Autodesk Fusion 360 part; units mm, degrees
(part 4 of 15)
  spline S55 degree 5 poles (25.1717, 7.6599) (25.182, 7.6631) (25.2028, 7.6691) (25.2341, 7.6774) (25.2761, 7.6871) (25.3292, 7.6971) (25.3826, 7.7058) (25.4363, 7.7136) (25.4901, 7.7209) (25.544, 7.7279) (25.598, 7.7346) (25.6521, 7.7408) (25.7063, 7.7465) (25.7606, 7.7514) (25.8152, 7.7557) (25.8698, 7.7594) (25.9246, 7.7625) (25.9795, 7.7651) (26.0345, 7.7673) (26.0895, 7.7692) (26.1446, 7.7706) (26.1998, 7.7717) (26.2551, 7.7724) (26.3104, 7.7726) (26.3659, 7.7725) (26.4214, 7.7719) (26.4769, 7.7709) (26.5326, 7.7695) (26.5883, 7.7678) (26.644, 7.7657) (26.6999, 7.7633) (26.7557, 7.7606) (26.8117, 7.7575) (26.8676, 7.754) (26.9237, 7.7502) (26.9797, 7.7461) (27.0359, 7.7417) (27.092, 7.7369) (27.1483, 7.7318) (27.2045, 7.7264) (27.2608, 7.7206) (27.3172, 7.7146) (27.3735, 7.7083) (27.4299, 7.7016) (27.4864, 7.6947) (27.5429, 7.6874) (27.5994, 7.6799) (27.6559, 7.672) (27.7125, 7.6639) (27.7691, 7.6555) (27.8257, 7.6468) (27.8824, 7.6378) (27.9391, 7.6285) (27.9958, 7.6189) (28.0525, 7.6091) (28.1093, 7.599) (28.166, 7.5886) (28.2228, 7.5779) (28.2796, 7.567) (28.3365, 7.5558) (28.3933, 7.5443) (28.4502, 7.5326) (28.5071, 7.5206) (28.564, 7.5083) (28.6209, 7.4958) (28.6778, 7.483) (28.7347, 7.47) (28.7917, 7.4567) (28.8486, 7.4431) (28.9056, 7.4293) (28.9625, 7.4152) (29.0081, 7.4038) (29.0423, 7.3951) (29.0651, 7.3892) (29.0765, 7.3863) knots 0 0 0 0 0 0 0.01428571 0.02857143 0.04285714 0.05714286 0.07142857 0.08571429 0.1 0.11428571 0.12857143 0.14285714 0.15714286 0.17142857 0.18571429 0.2 0.21428571 0.22857143 0.24285714 0.25714286 0.27142857 0.28571429 0.3 0.31428571 0.32857143 0.34285714 0.35714286 0.37142857 0.38571429 0.4 0.41428571 0.42857143 0.44285714 0.45714286 0.47142857 0.48571429 0.5 0.51428571 0.52857143 0.54285714 0.55714286 0.57142857 0.58571429 0.6 0.61428571 0.62857143 0.64285714 0.65714286 0.67142857 0.68571429 0.7 0.71428571 0.72857143 0.74285714 0.75714286 0.77142857 0.78571429 0.8 0.81428571 0.82857143 0.84285714 0.85714286 0.87142857 0.88571429 0.9 0.91428571 0.92857143 0.94285714 0.95714286 0.97142857 0.98571429 1 1 1 1 1 1
  line L55 (25.1717, 7.6599) -> (24.5734, 7.4779)
  circle A57 centre (0, 0) radius 20
  dimension "d90" = 40
  constraint concentric A0 A57
  measures "d90" diameter of A57
extrude "Extrude3'" add sketch "Sketch4" along normal blind 40 contours A0 | A57 bodies 9 in component "Spur Gear 28 teeth"
hole "Hole1" at (0, 20, -27.403) direction (0, -1, 0) diameter 8 end through all bodies 9 in component "Spur Gear 28 teeth"
pattern_circular "C-Pattern2" count 3 over 360 about axis through (0, 0, -40) along (0, 0, -1) of "Hole1" in component "Spur Gear 28 teeth"
sketch "Base Circle (3)" plane through (0, 0, 0) normal (0, 0, 1) x (1, 0, 0) in component "Spur Gear 88 teeth"
  circle A0 centre (0, 0) radius 68.5488
  circle A1 centre (0, 0) radius 10
extrude "Extrude1''''" add sketch "Base Circle (3)" along normal blind 20 separate body makes body 10 in component "Spur Gear 88 teeth"
sketch "Gear Tooth (3)" plane through (0, 0, 0) normal (0, 0, 1) x (1, 0, 0) in component "Spur Gear 88 teeth"
  spline S0 degree 5 poles (66.1189, -2.1665) (66.1359, -2.1663) (66.1698, -2.166) (66.2208, -2.1651) (66.2887, -2.1631) (66.3736, -2.1595) (66.4585, -2.1546) (66.5434, -2.1486) (66.6283, -2.1414) (66.7132, -2.1332) (66.7981, -2.1241) (66.8829, -2.1141) (66.9678, -2.1035) (67.0526, -2.0922) (67.1374, -2.0802) (67.2222, -2.0677) (67.3069, -2.0546) (67.3917, -2.0409) (67.4764, -2.0267) (67.561, -2.0118) (67.6457, -1.9964) (67.7303, -1.9805) (67.8149, -1.964) (67.8995, -1.9471) (67.984, -1.9297) (68.0685, -1.9118) (68.153, -1.8935) (68.2374, -1.8747) (68.3218, -1.8554) (68.4062, -1.8357) (68.4905, -1.8156) (68.5748, -1.795) (68.6591, -1.774) (68.7433, -1.7526) (68.8275, -1.7308) (68.9117, -1.7086) (68.9958, -1.686) (69.0799, -1.6631) (69.164, -1.6397) (69.248, -1.6159) (69.332, -1.5918) (69.4159, -1.5673) (69.4999, -1.5425) (69.5837, -1.5172) (69.6675, -1.4917) (69.7513, -1.4657) (69.8351, -1.4394) (69.9188, -1.4128) (70.0025, -1.3858) (70.0861, -1.3585) (70.1697, -1.3308) (70.2532, -1.3028) (70.3367, -1.2745) (70.4201, -1.2458) (70.5036, -1.2169) (70.5869, -1.1876) (70.6703, -1.1579) (70.7535, -1.128) (70.8368, -1.0977) (70.92, -1.0672) (71.0031, -1.0363) (71.0862, -1.0051) (71.1692, -0.9736) (71.2522, -0.9418) (71.3352, -0.9097) (71.4181, -0.8773) (71.501, -0.8446) (71.5838, -0.8116) (71.6666, -0.7783) (71.7493, -0.7447) (71.832, -0.7108) (71.8981, -0.6835) (71.9476, -0.6629) (71.9806, -0.649) (71.9971, -0.6421) knots 0 0 0 0 0 0 0.01428571 0.02857143 0.04285714 0.05714286 0.07142857 0.08571429 0.1 0.11428571 0.12857143 0.14285714 0.15714286 0.17142857 0.18571429 0.2 0.21428571 0.22857143 0.24285714 0.25714286 0.27142857 0.28571429 0.3 0.31428571 0.32857143 0.34285714 0.35714286 0.37142857 0.38571429 0.4 0.41428571 0.42857143 0.44285714 0.45714286 0.47142857 0.48571429 0.5 0.51428571 0.52857143 0.54285714 0.55714286 0.57142857 0.58571429 0.6 0.61428571 0.62857143 0.64285714 0.65714286 0.67142857 0.68571429 0.7 0.71428571 0.72857143 0.74285714 0.75714286 0.77142857 0.78571429 0.8 0.81428571 0.82857143 0.84285714 0.85714286 0.87142857 0.88571429 0.9 0.91428571 0.92857143 0.94285714 0.95714286 0.97142857 0.98571429 1 1 1 1 1 1
  spline S1 degree 5 poles (66.1189, 2.1665) (66.1359, 2.1663) (66.1698, 2.166) (66.2208, 2.1651) (66.2887, 2.1631) (66.3736, 2.1595) (66.4585, 2.1546) (66.5434, 2.1486) (66.6283, 2.1414) (66.7132, 2.1332) (66.7981, 2.1241) (66.8829, 2.1141) (66.9678, 2.1035) (67.0526, 2.0922) (67.1374, 2.0802) (67.2222, 2.0677) (67.3069, 2.0546) (67.3917, 2.0409) (67.4764, 2.0267) (67.561, 2.0118) (67.6457, 1.9964) (67.7303, 1.9805) (67.8149, 1.964) (67.8995, 1.9471) (67.984, 1.9297) (68.0685, 1.9118) (68.153, 1.8935) (68.2374, 1.8747) (68.3218, 1.8554) (68.4062, 1.8357) (68.4905, 1.8156) (68.5748, 1.795) (68.6591, 1.774) (68.7433, 1.7526) (68.8275, 1.7308) (68.9117, 1.7086) (68.9958, 1.686) (69.0799, 1.6631) (69.164, 1.6397) (69.248, 1.6159) (69.332, 1.5918) (69.4159, 1.5673) (69.4999, 1.5425) (69.5837, 1.5172) (69.6675, 1.4917) (69.7513, 1.4657) (69.8351, 1.4394) (69.9188, 1.4128) (70.0025, 1.3858) (70.0861, 1.3585) (70.1697, 1.3308) (70.2532, 1.3028) (70.3367, 1.2745) (70.4201, 1.2458) (70.5036, 1.2169) (70.5869, 1.1876) (70.6703, 1.1579) (70.7535, 1.128) (70.8368, 1.0977) (70.92, 1.0672) (71.0031, 1.0363) (71.0862, 1.0051) (71.1692, 0.9736) (71.2522, 0.9418) (71.3352, 0.9097) (71.4181, 0.8773) (71.501, 0.8446) (71.5838, 0.8116) (71.6666, 0.7783) (71.7493, 0.7447) (71.832, 0.7108) (71.8981, 0.6835) (71.9476, 0.6629) (71.9806, 0.649) (71.9971, 0.6421) knots 0 0 0 0 0 0 0.01428571 0.02857143 0.04285714 0.05714286 0.07142857 0.08571429 0.1 0.11428571 0.12857143 0.14285714 0.15714286 0.17142857 0.18571429 0.2 0.21428571 0.22857143 0.24285714 0.25714286 0.27142857 0.28571429 0.3 0.31428571 0.32857143 0.34285714 0.35714286 0.37142857 0.38571429 0.4 0.41428571 0.42857143 0.44285714 0.45714286 0.47142857 0.48571429 0.5 0.51428571 0.52857143 0.54285714 0.55714286 0.57142857 0.58571429 0.6 0.61428571 0.62857143 0.64285714 0.65714286 0.67142857 0.68571429 0.7 0.71428571 0.72857143 0.74285714 0.75714286 0.77142857 0.78571429 0.8 0.81428571 0.82857143 0.84285714 0.85714286 0.87142857 0.88571429 0.9 0.91428571 0.92857143 0.94285714 0.95714286 0.97142857 0.98571429 1 1 1 1 1 1
  arc A0 (71.9971, -0.6421) -> (71.9971, 0.6421) centre (0, 0) ccw
  line L0 (66.1189, 2.1665) -> (66.1189, -2.1665)
  point P0 (66.5372, -2.1488)
  point P1 (66.9564, -2.1048)
  point P2 (67.376, -2.0434)
  point P3 (67.796, -1.9676)
  point P4 (68.2162, -1.8793)
  point P5 (68.6366, -1.7796)
  point P6 (69.057, -1.6693)
  point P7 (69.4775, -1.549)
  point P8 (69.8979, -1.4194)
  point P9 (70.3182, -1.2807)
  point P10 (70.7383, -1.1334)
  point P11 (71.1582, -0.9777)
  point P12 (71.5778, -0.8139)
  point P13 (66.5372, 2.1488)
  point P14 (66.9564, 2.1048)
  point P15 (67.376, 2.0434)
  point P16 (67.796, 1.9676)
  point P17 (68.2162, 1.8793)
  point P18 (68.6366, 1.7796)
  point P19 (69.057, 1.6693)
  point P20 (69.4775, 1.549)
  point P21 (69.8979, 1.4194)
  point P22 (70.3182, 1.2807)
  point P23 (70.7383, 1.1334)
  point P24 (71.1582, 0.9777)
  point P25 (71.5778, 0.8139)
extrude "Extrude2''''" add sketch "Gear Tooth (3)" along normal blind 20 bodies 10 in component "Spur Gear 88 teeth"
pattern_circular "C-Pattern1''" count 88 over 360 about axis through (0, 0, 0) along (0, 0, 1) of "Extrude2''''" in component "Spur Gear 88 teeth"
sketch "Diametrial Pitch Circle (3)" plane through (0, 0, 0) normal (0, 0, 1) x (1, 0, 0) in component "Spur Gear 88 teeth"
  circle A0 centre (0, 0) radius 70.4 construction
scale "Scale1" factor 1.03 about (35.5272, 58.6239, 20) bodies 10 in component "Spur Gear 88 teeth"
sketch "Sketch1 (3)" plane through (0, 173.8907, 0) normal (0, -1, 0) x (1, 0, 0) in component "Base2"
  arc A0 (68.5305, -56.0481) -> (68.5775, -54.7308) centre (-2.0032, -52.8695) ccw
  spline S0 degree 5 poles (68.5775, -54.7308) (68.5878, -54.7283) (68.6154, -54.7216) (68.6604, -54.7105) (68.7228, -54.6949) (68.8024, -54.6747) (68.8892, -54.6522) (68.9759, -54.6294) (69.0625, -54.6061) (69.1491, -54.5824) (69.2357, -54.5584) (69.3222, -54.5339) (69.4087, -54.5091) (69.4952, -54.4838) (69.5816, -54.4582) (69.668, -54.4322) (69.7544, -54.4059) (69.8407, -54.3792) (69.9269, -54.3521) (70.0131, -54.3247) (70.0993, -54.2969) (70.1854, -54.2687) (70.2715, -54.2402) (70.3576, -54.2114) (70.4436, -54.1822) (70.5295, -54.1527) (70.6155, -54.1228) (70.7013, -54.0927) (70.7871, -54.0621) (70.8729, -54.0313) (70.9587, -54.0001) (71.0443, -53.9686) (71.13, -53.9368) (71.2156, -53.9047) (71.3011, -53.8723) (71.3866, -53.8395) (71.472, -53.8064) (71.5574, -53.7731) (71.6428, -53.7394) (71.7281, -53.7054) (71.8133, -53.6711) (71.8985, -53.6365) (71.9837, -53.6016) (72.0518, -53.5735) (72.1028, -53.5522) (72.1368, -53.538) (72.1538, -53.5309) knots 0.405839 0.405839 0.405839 0.405839 0.405839 0.405839 0.414286 0.428571 0.442857 0.457143 0.471429 0.485714 0.5 0.514286 0.528571 0.542857 0.557143 0.571429 0.585714 0.6 0.614286 0.628571 0.642857 0.657143 0.671429 0.685714 0.7 0.714286 0.728571 0.742857 0.757143 0.771429 0.785714 0.8 0.814286 0.828571 0.842857 0.857143 0.871429 0.885714 0.9 0.914286 0.928571 0.942857 0.957143 0.971429 0.985714 1 1 1 1 1 1
  arc A1 (72.1538, -53.5309) -> (72.1538, -52.2081) centre (-2.0032, -52.8695) ccw
  spline S1 degree 5 poles (72.1538, -52.2081) (72.1368, -52.201) (72.1028, -52.1867) (72.0518, -52.1655) (71.9837, -52.1373) (71.8985, -52.1025) (71.8133, -52.0679) (71.7281, -52.0336) (71.6428, -51.9996) (71.5574, -51.9659) (71.472, -51.9325) (71.3866, -51.8995) (71.3011, -51.8667) (71.2156, -51.8343) (71.13, -51.8021) (71.0443, -51.7703) (70.9587, -51.7388) (70.8729, -51.7077) (70.7871, -51.6768) (70.7013, -51.6463) (70.6155, -51.6161) (70.5295, -51.5863) (70.4436, -51.5567) (70.3576, -51.5276) (70.2715, -51.4987) (70.1854, -51.4702) (70.0993, -51.4421) (70.0131, -51.4143) (69.9269, -51.3869) (69.8407, -51.3598) (69.7544, -51.3331) (69.668, -51.3067) (69.5816, -51.2807) (69.4952, -51.2551) (69.4087, -51.2299) (69.3222, -51.2051) (69.2357, -51.1806) (69.1491, -51.1565) (69.0625, -51.1329) (68.9759, -51.1096) (68.8892, -51.0867) (68.8024, -51.0643) (68.7228, -51.044) (68.6604, -51.0285) (68.6154, -51.0174) (68.5878, -51.0107) (68.5775, -51.0082) knots -1 -1 -1 -1 -1 -1 -0.985714 -0.971429 -0.957143 -0.942857 -0.928571 -0.914286 -0.9 -0.885714 -0.871429 -0.857143 -0.842857 -0.828571 -0.814286 -0.8 -0.785714 -0.771429 -0.757143 -0.742857 -0.728571 -0.714286 -0.7 -0.685714 -0.671429 -0.657143 -0.642857 -0.628571 -0.614286 -0.6 -0.585714 -0.571429 -0.557143 -0.542857 -0.528571 -0.514286 -0.5 -0.485714 -0.471429 -0.457143 -0.442857 -0.428571 -0.414286 -0.405839 -0.405839 -0.405839 -0.405839 -0.405839 -0.405839
  arc A2 (68.5775, -51.0082) -> (68.5305, -49.6909) centre (-2.0032, -52.8695) ccw
  spline S2 degree 5 poles (68.5305, -49.6909) (68.5405, -49.6877) (68.5676, -49.679) (68.6117, -49.6647) (68.6728, -49.6447) (68.7508, -49.6189) (68.8357, -49.5903) (68.9206, -49.5613) (69.0053, -49.5319) (69.09, -49.5021) (69.1747, -49.4719) (69.2593, -49.4414) (69.3438, -49.4104) (69.4282, -49.3791) (69.5126, -49.3474) (69.5969, -49.3153) (69.6811, -49.2828) (69.7653, -49.25) (69.8494, -49.2169) (69.9335, -49.1834) (70.0174, -49.1495) (70.1013, -49.1153) (70.1852, -49.0807) (70.2689, -49.0458) (70.3526, -49.0106) (70.4363, -48.975) (70.5198, -48.9391) (70.6033, -48.9029) (70.6868, -48.8663) (70.7701, -48.8294) (70.8534, -48.7922) (70.9366, -48.7547) (71.0198, -48.7169) (71.1029, -48.6787) (71.1859, -48.6402) (71.2688, -48.6015) (71.3517, -48.5624) (71.4345, -48.523) (71.5172, -48.4833) (71.5999, -48.4433) (71.6825, -48.403) (71.765, -48.3625) (71.8474, -48.3216) (71.9133, -48.2887) (71.9627, -48.2638) (71.9956, -48.2472) (72.0121, -48.2389) knots 0.405839 0.405839 0.405839 0.405839 0.405839 0.405839 0.414286 0.428571 0.442857 0.457143 0.471429 0.485714 0.5 0.514286 0.528571 0.542857 0.557143 0.571429 0.585714 0.6 0.614286 0.628571 0.642857 0.657143 0.671429 0.685714 0.7 0.714286 0.728571 0.742857 0.757143 0.771429 0.785714 0.8 0.814286 0.828571 0.842857 0.857143 0.871429 0.885714 0.9 0.914286 0.928571 0.942857 0.957143 0.971429 0.985714 1 1 1 1 1 1
  arc A3 (72.0121, -48.2389) -> (71.9177, -46.9195) centre (-2.0032, -52.8695) ccw
  spline S3 degree 5 poles (71.9177, -46.9195) (71.9002, -46.9136) (71.8653, -46.9018) (71.8129, -46.8843) (71.743, -46.861) (71.6555, -46.8323) (71.5681, -46.8039) (71.4806, -46.7758) (71.3931, -46.748) (71.3056, -46.7204) (71.218, -46.6932) (71.1304, -46.6664) (71.0428, -46.6398) (70.9552, -46.6135) (70.8675, -46.5876) (70.7798, -46.562) (70.6921, -46.5367) (70.6044, -46.5117) (70.5166, -46.487) (70.4288, -46.4627) (70.341, -46.4387) (70.2532, -46.4151) (70.1653, -46.3918) (70.0775, -46.3688) (69.9896, -46.3462) (69.9017, -46.3239) (69.8138, -46.302) (69.7258, -46.2804) (69.6379, -46.2592) (69.5499, -46.2384) (69.4619, -46.2179) (69.3739, -46.1977) (69.2859, -46.178) (69.1979, -46.1586) (69.1098, -46.1396) (69.0218, -46.121) (68.9337, -46.1028) (68.8456, -46.0849) (68.7576, -46.0675) (68.6695, -46.0505) (68.5814, -46.0339) (68.4932, -46.0177) (68.4123, -46.0032) (68.349, -45.9921) (68.3034, -45.9843) (68.2753, -45.9795) (68.2649, -45.9777) knots -1 -1 -1 -1 -1 -1 -0.985714 -0.971429 -0.957143 -0.942857 -0.928571 -0.914286 -0.9 -0.885714 -0.871429 -0.857143 -0.842857 -0.828571 -0.814286 -0.8 -0.785714 -0.771429 -0.757143 -0.742857 -0.728571 -0.714286 -0.7 -0.685714 -0.671429 -0.657143 -0.642857 -0.628571 -0.614286 -0.6 -0.585714 -0.571429 -0.557143 -0.542857 -0.528571 -0.514286 -0.5 -0.485714 -0.471429 -0.457143 -0.442857 -0.428571 -0.414286 -0.405839 -0.405839 -0.405839 -0.405839 -0.405839 -0.405839
  arc A4 (68.2649, -45.9777) -> (68.124, -44.6672) centre (-2.0032, -52.8695) ccw
  spline S4 degree 5 poles (68.124, -44.6672) (68.1338, -44.6632) (68.1602, -44.6526) (68.2032, -44.6353) (68.2627, -44.611) (68.3386, -44.5796) (68.4213, -44.5451) (68.5038, -44.5101) (68.5863, -44.4747) (68.6687, -44.439) (68.7509, -44.4028) (68.8331, -44.3663) (68.9152, -44.3294) (68.9972, -44.2921) (69.0791, -44.2545) (69.1609, -44.2165) (69.2426, -44.1781) (69.3242, -44.1394) (69.4058, -44.1003) (69.4872, -44.0608) (69.5686, -44.0211) (69.6498, -43.981) (69.731, -43.9405) (69.812, -43.8997) (69.893, -43.8586) (69.9739, -43.8172) (70.0547, -43.7754) (70.1354, -43.7333) (70.216, -43.6909) (70.2965, -43.6481) (70.3769, -43.6051) (70.4572, -43.5617) (70.5375, -43.518) (70.6176, -43.4741) (70.6977, -43.4298) (70.7776, -43.3852) (70.8575, -43.3403) (70.9373, -43.2951) (71.017, -43.2496) (71.0966, -43.2038) (71.1761, -43.1577) (71.2555, -43.1114) (71.3348, -43.0647) (71.3982, -43.0272) (71.4457, -42.9989) (71.4773, -42.98) (71.4932, -42.9705) knots 0.405839 0.405839 0.405839 0.405839 0.405839 0.405839 0.414286 0.428571 0.442857 0.457143 0.471429 0.485714 0.5 0.514286 0.528571 0.542857 0.557143 0.571429 0.585714 0.6 0.614286 0.628571 0.642857 0.657143 0.671429 0.685714 0.7 0.714286 0.728571 0.742857 0.757143 0.771429 0.785714 0.8 0.814286 0.828571 0.842857 0.857143 0.871429 0.885714 0.9 0.914286 0.928571 0.942857 0.957143 0.971429 0.985714 1 1 1 1 1 1
  arc A5 (71.4932, -42.9705) -> (71.3049, -41.6612) centre (-2.0032, -52.8695) ccw
  spline S5 degree 5 poles (71.3049, -41.6612) (71.2871, -41.6565) (71.2514, -41.6473) (71.1978, -41.6335) (71.1264, -41.6154) (71.0372, -41.5929) (70.9479, -41.5708) (70.8587, -41.549) (70.7694, -41.5275) (70.6801, -41.5063) (70.5908, -41.4854) (70.5016, -41.4649) (70.4123, -41.4446) (70.323, -41.4247) (70.2337, -41.4051) (70.1444, -41.3858) (70.0551, -41.3668) (69.9658, -41.3481) (69.8765, -41.3298) (69.7872, -41.3118) (69.6979, -41.2942) (69.6086, -41.2768) (69.5194, -41.2599) (69.4301, -41.2432) (69.3408, -41.2269) (69.2515, -41.211) (69.1623, -41.1954) (69.073, -41.1801) (68.9838, -41.1652) (68.8945, -41.1507) (68.8053, -41.1365) (68.7161, -41.1227) (68.6269, -41.1093) (68.5377, -41.0963) (68.4485, -41.0836) (68.3594, -41.0713) (68.2702, -41.0594) (68.1811, -41.0479) (68.092, -41.0368) (68.0029, -41.0261) (67.9139, -41.0158) (67.8248, -41.006) (67.7431, -40.9973) (67.6792, -40.9907) (67.633, -40.9862) (67.6047, -40.9834) (67.5942, -40.9824) knots -1 -1 -1 -1 -1 -1 -0.985714 -0.971429 -0.957143 -0.942857 -0.928571 -0.914286 -0.9 -0.885714 -0.871429 -0.857143 -0.842857 -0.828571 -0.814286 -0.8 -0.785714 -0.771429 -0.757143 -0.742857 -0.728571 -0.714286 -0.7 -0.685714 -0.671429 -0.657143 -0.642857 -0.628571 -0.614286 -0.6 -0.585714 -0.571429 -0.557143 -0.542857 -0.528571 -0.514286 -0.5 -0.485714 -0.471429 -0.457143 -0.442857 -0.428571 -0.414286 -0.405839 -0.405839 -0.405839 -0.405839 -0.405839 -0.405839
  arc A6 (67.5942, -40.9824) -> (67.3602, -39.6853) centre (-2.0032, -52.8695) ccw
  spline S6 degree 5 poles (67.3602, -39.6853) (67.3697, -39.6806) (67.3952, -39.6682) (67.4369, -39.6478) (67.4945, -39.6193) (67.568, -39.5826) (67.648, -39.5422) (67.7279, -39.5015) (67.8076, -39.4603) (67.8872, -39.4188) (67.9667, -39.3769) (68.046, -39.3346) (68.1253, -39.2919) (68.2044, -39.2489) (68.2834, -39.2055) (68.3623, -39.1617) (68.4411, -39.1176) (68.5197, -39.0732) (68.5982, -39.0284) (68.6767, -38.9832) (68.755, -38.9377) (68.8331, -38.8919) (68.9112, -38.8458) (68.9892, -38.7993) (69.067, -38.7525) (69.1447, -38.7054) (69.2223, -38.658) (69.2998, -38.6102) (69.3772, -38.5622) (69.4544, -38.5138) (69.5316, -38.4651) (69.6086, -38.4162) (69.6855, -38.3669) (69.7623, -38.3173) (69.839, -38.2674) (69.9156, -38.2172) (69.9921, -38.1667) (70.0684, -38.116) (70.1447, -38.0649) (70.2208, -38.0136) (70.2968, -37.9619) (70.3727, -37.91) (70.4485, -37.8578) (70.509, -37.8159) (70.5544, -37.7842) (70.5846, -37.7631) (70.5997, -37.7525) knots 0.405839 0.405839 0.405839 0.405839 0.405839 0.405839 0.414286 0.428571 0.442857 0.457143 0.471429 0.485714 0.5 0.514286 0.528571 0.542857 0.557143 0.571429 0.585714 0.6 0.614286 0.628571 0.642857 0.657143 0.671429 0.685714 0.7 0.714286 0.728571 0.742857 0.757143 0.771429 0.785714 0.8 0.814286 0.828571 0.842857 0.857143 0.871429 0.885714 0.9 0.914286 0.928571 0.942857 0.957143 0.971429 0.985714 1 1 1 1 1 1
  arc A7 (70.5997, -37.7525) -> (70.3185, -36.46) centre (-2.0032, -52.8695) ccw
  spline S7 degree 5 poles (70.3185, -36.46) (70.3004, -36.4566) (70.2641, -36.45) (70.2097, -36.4401) (70.1372, -36.427) (70.0466, -36.411) (69.956, -36.3953) (69.8654, -36.38) (69.7748, -36.3649) (69.6843, -36.3501) (69.5937, -36.3356) (69.5032, -36.3215) (69.4127, -36.3077) (69.3222, -36.2941) (69.2318, -36.2809) (69.1413, -36.2681) (69.0509, -36.2555) (68.9605, -36.2433) (68.8701, -36.2314) (68.7798, -36.2198) (68.6895, -36.2085) (68.5992, -36.1976) (68.5089, -36.1871) (68.4187, -36.1768) (68.3285, -36.167) (68.2383, -36.1574) (68.1481, -36.1482) (68.058, -36.1394) (67.9679, -36.1309) (67.8779, -36.1228) (67.7879, -36.115) (67.6979, -36.1076) (67.608, -36.1006) (67.5181, -36.0939) (67.4282, -36.0877) (67.3384, -36.0818) (67.2487, -36.0763) (67.159, -36.0712) (67.0693, -36.0664) (66.9797, -36.0621) (66.8901, -36.0582) (66.8006, -36.0547) (66.7184, -36.0519) (66.6542, -36.0499) (66.6079, -36.0487) (66.5794, -36.0479) (66.5689, -36.0477) knots -1 -1 -1 -1 -1 -1 -0.985714 -0.971429 -0.957143 -0.942857 -0.928571 -0.914286 -0.9 -0.885714 -0.871429 -0.857143 -0.842857 -0.828571 -0.814286 -0.8 -0.785714 -0.771429 -0.757143 -0.742857 -0.728571 -0.714286 -0.7 -0.685714 -0.671429 -0.657143 -0.642857 -0.628571 -0.614286 -0.6 -0.585714 -0.571429 -0.557143 -0.542857 -0.528571 -0.514286 -0.5 -0.485714 -0.471429 -0.457143 -0.442857 -0.428571 -0.414286 -0.405839 -0.405839 -0.405839 -0.405839 -0.405839 -0.405839
  arc A8 (66.5689, -36.0477) -> (66.2429, -34.7705) centre (-2.0032, -52.8695) ccw
  spline S8 degree 5 poles (66.2429, -34.7705) (66.252, -34.7652) (66.2767, -34.751) (66.3167, -34.7277) (66.3721, -34.6952) (66.4429, -34.6533) (66.5198, -34.6073) (66.5965, -34.561) (66.6731, -34.5142) (66.7496, -34.4671) (66.8258, -34.4196) (66.902, -34.3718) (66.978, -34.3236) (67.0538, -34.275) (67.1295, -34.2261) (67.2051, -34.1768) (67.2805, -34.1272) (67.3558, -34.0773) (67.4309, -34.027) (67.5059, -33.9764) (67.5808, -33.9254) (67.6555, -33.8741) (67.7301, -33.8226) (67.8045, -33.7706) (67.8788, -33.7184) (67.953, -33.6659) (68.027, -33.613) (68.1009, -33.5599) (68.1746, -33.5064) (68.2482, -33.4527) (68.3217, -33.3986) (68.3951, -33.3442) (68.4683, -33.2896) (68.5413, -33.2347) (68.6143, -33.1794) (68.6871, -33.1239) (68.7598, -33.0681) (68.8323, -33.012) (68.9047, -32.9557) (68.977, -32.899) (69.0491, -32.8421) (69.1211, -32.7849) (69.193, -32.7274) (69.2504, -32.6812) (69.2934, -32.6465) (69.322, -32.6233) (69.3363, -32.6116) knots 0.405839 0.405839 0.405839 0.405839 0.405839 0.405839 0.414286 0.428571 0.442857 0.457143 0.471429 0.485714 0.5 0.514286 0.528571 0.542857 0.557143 0.571429 0.585714 0.6 0.614286 0.628571 0.642857 0.657143 0.671429 0.685714 0.7 0.714286 0.728571 0.742857 0.757143 0.771429 0.785714 0.8 0.814286 0.828571 0.842857 0.857143 0.871429 0.885714 0.9 0.914286 0.928571 0.942857 0.957143 0.971429 0.985714 1 1 1 1 1 1
  arc A9 (69.3363, -32.6116) -> (68.9636, -31.3424) centre (-2.0032, -52.8695) ccw
  spline S9 degree 5 poles (68.9636, -31.3424) (68.9453, -31.3404) (68.9087, -31.3363) (68.8537, -31.3303) (68.7804, -31.3225) (68.6889, -31.313) (68.5974, -31.3038) (68.506, -31.2949) (68.4145, -31.2863) (68.3232, -31.2781) (68.2318, -31.2701) (68.1405, -31.2624) (68.0493, -31.2551) (67.958, -31.2481) (67.8669, -31.2414) (67.7757, -31.235) (67.6846, -31.2289) (67.5936, -31.2231) (67.5026, -31.2177) (67.4117, -31.2126) (67.3208, -31.2078) (67.2299, -31.2034) (67.1391, -31.1993) (67.0484, -31.1955) (66.9577, -31.1921) (66.8671, -31.189) (66.7765, -31.1863) (66.686, -31.1839) (66.5955, -31.1819) (66.5052, -31.1802) (66.4148, -31.1789) (66.3246, -31.1779) (66.2343, -31.1773) (66.1442, -31.1771) (66.0541, -31.1772) (65.9641, -31.1778) (65.8742, -31.1787) (65.7844, -31.18) (65.6946, -31.1817) (65.6049, -31.1838) (65.5153, -31.1862) (65.4257, -31.1891) (65.3436, -31.1922) (65.2794, -31.1948) (65.2331, -31.1969) (65.2047, -31.1982) (65.1941, -31.1987) knots -1 -1 -1 -1 -1 -1 -0.985714 -0.971429 -0.957143 -0.942857 -0.928571 -0.914286 -0.9 -0.885714 -0.871429 -0.857143 -0.842857 -0.828571 -0.814286 -0.8 -0.785714 -0.771429 -0.757143 -0.742857 -0.728571 -0.714286 -0.7 -0.685714 -0.671429 -0.657143 -0.642857 -0.628571 -0.614286 -0.6 -0.585714 -0.571429 -0.557143 -0.542857 -0.528571 -0.514286 -0.5 -0.485714 -0.471429 -0.457143 -0.442857 -0.428571 -0.414286 -0.405839 -0.405839 -0.405839 -0.405839 -0.405839 -0.405839
  arc A10 (65.1941, -31.1987) -> (64.7778, -29.948) centre (-2.0032, -52.8695) ccw
  spline S10 degree 5 poles (64.7778, -29.948) (64.7866, -29.9421) (64.8101, -29.9261) (64.8484, -29.9) (64.9014, -29.8636) (64.969, -29.8168) (65.0424, -29.7655) (65.1156, -29.7138) (65.1887, -29.6617) (65.2616, -29.6092) (65.3343, -29.5564) (65.4068, -29.5033) (65.4792, -29.4498) (65.5514, -29.3959) (65.6234, -29.3417) (65.6953, -29.2872) (65.7669, -29.2323) (65.8385, -29.1771) (65.9098, -29.1216) (65.981, -29.0658) (66.052, -29.0096) (66.1229, -28.9531) (66.1936, -28.8964) (66.2642, -28.8393) (66.3345, -28.7819) (66.4048, -28.7242) (66.4748, -28.6662) (66.5447, -28.6079) (66.6145, -28.5493) (66.6841, -28.4905) (66.7535, -28.4313) (66.8228, -28.3718) (66.8919, -28.3121) (66.9609, -28.2521) (67.0297, -28.1918) (67.0983, -28.1312) (67.1668, -28.0704) (67.2352, -28.0093) (67.3034, -27.9479) (67.3714, -27.8862) (67.4393, -27.8243) (67.5071, -27.7621) (67.5747, -27.6997) (67.6286, -27.6495) (67.669, -27.6118) (67.6959, -27.5866) (67.7093, -27.5739) knots 0.405839 0.405839 0.405839 0.405839 0.405839 0.405839 0.414286 0.428571 0.442857 0.457143 0.471429 0.485714 0.5 0.514286 0.528571 0.542857 0.557143 0.571429 0.585714 0.6 0.614286 0.628571 0.642857 0.657143 0.671429 0.685714 0.7 0.714286 0.728571 0.742857 0.757143 0.771429 0.785714 0.8 0.814286 0.828571 0.842857 0.857143 0.871429 0.885714 0.9 0.914286 0.928571 0.942857 0.957143 0.971429 0.985714 1 1 1 1 1 1
  arc A11 (67.7093, -27.5739) -> (67.2471, -26.3346) centre (-2.0032, -52.8695) ccw
  spline S11 degree 5 poles (67.2471, -26.3346) (67.2287, -26.3338) (67.1918, -26.3324) (67.1366, -26.3303) (67.0629, -26.3277) (66.971, -26.3248) (66.8791, -26.3222) (66.7872, -26.3198) (66.6954, -26.3178) (66.6037, -26.3161) (66.512, -26.3146) (66.4204, -26.3135) (66.3288, -26.3127) (66.2373, -26.3122) (66.1459, -26.312) (66.0545, -26.3121) (65.9633, -26.3126) (65.872, -26.3133) (65.7809, -26.3144) (65.6898, -26.3158) (65.5988, -26.3175) (65.5079, -26.3196) (65.417, -26.322) (65.3263, -26.3247) (65.2356, -26.3277) (65.1449, -26.3311) (65.0544, -26.3348) (64.964, -26.3389) (64.8736, -26.3433) (64.7833, -26.3481) (64.6931, -26.3532) (64.603, -26.3587) (64.513, -26.3646) (64.4231, -26.3708) (64.3332, -26.3774) (64.2435, -26.3843) (64.1539, -26.3916) (64.0643, -26.3993) (63.9749, -26.4074) (63.8856, -26.4159) (63.7964, -26.4248) (63.7073, -26.4341) (63.6255, -26.4429) (63.5617, -26.4502) (63.5157, -26.4555) (63.4874, -26.4588) (63.4769, -26.4601) knots -1 -1 -1 -1 -1 -1 -0.985714 -0.971429 -0.957143 -0.942857 -0.928571 -0.914286 -0.9 -0.885714 -0.871429 -0.857143 -0.842857 -0.828571 -0.814286 -0.8 -0.785714 -0.771429 -0.757143 -0.742857 -0.728571 -0.714286 -0.7 -0.685714 -0.671429 -0.657143 -0.642857 -0.628571 -0.614286 -0.6 -0.585714 -0.571429 -0.557143 -0.542857 -0.528571 -0.514286 -0.5 -0.485714 -0.471429 -0.457143 -0.442857 -0.428571 -0.414286 -0.405839 -0.405839 -0.405839 -0.405839 -0.405839 -0.405839
  arc A12 (63.4769, -26.4601) -> (62.9725, -25.2423) centre (-2.0032, -52.8695) ccw
  spline S12 degree 5 poles (62.9725, -25.2423) (62.9808, -25.2358) (63.0031, -25.2181) (63.0395, -25.1894) (63.0897, -25.1493) (63.1538, -25.0978) (63.2233, -25.0414) (63.2927, -24.9846) (63.3619, -24.9274) (63.4308, -24.8699) (63.4996, -24.812) (63.5681, -24.7538) (63.6365, -24.6953) (63.7047, -24.6364) (63.7726, -24.5772) (63.8404, -24.5177) (63.908, -24.4579) (63.9754, -24.3977) (64.0426, -24.3373) (64.1097, -24.2765) (64.1765, -24.2154) (64.2432, -24.154) (64.3096, -24.0923) (64.3759, -24.0304) (64.442, -23.9681) (64.508, -23.9055) (64.5737, -23.8427) (64.6393, -23.7796) (64.7047, -23.7162) (64.7699, -23.6525) (64.8349, -23.5885) (64.8998, -23.5243) (64.9645, -23.4598) (65.029, -23.395) (65.0933, -23.3299) (65.1575, -23.2646) (65.2215, -23.199) (65.2853, -23.1332) (65.3489, -23.0671) (65.4124, -23.0008) (65.4757, -22.9341) (65.5388, -22.8673) (65.6018, -22.8002) (65.652, -22.7463) (65.6896, -22.7058) (65.7147, -22.6787) (65.7272, -22.6651) knots 0.405839 0.405839 0.405839 0.405839 0.405839 0.405839 0.414286 0.428571 0.442857 0.457143 0.471429 0.485714 0.5 0.514286 0.528571 0.542857 0.557143 0.571429 0.585714 0.6 0.614286 0.628571 0.642857 0.657143 0.671429 0.685714 0.7 0.714286 0.728571 0.742857 0.757143 0.771429 0.785714 0.8 0.814286 0.828571 0.842857 0.857143 0.871429 0.885714 0.9 0.914286 0.928571 0.942857 0.957143 0.971429 0.985714 1 1 1 1 1 1
  arc A13 (65.7272, -22.6651) -> (65.1777, -21.4619) centre (-2.0032, -52.8695) ccw
  spline S13 degree 5 poles (65.1777, -21.4619) (65.1592, -21.4625) (65.1224, -21.4637) (65.0671, -21.4656) (64.9935, -21.4682) (64.9016, -21.4719) (64.8097, -21.4758) (64.7179, -21.48) (64.6262, -21.4845) (64.5346, -21.4894) (64.443, -21.4945) (64.3515, -21.4999) (64.2602, -21.5056) (64.1689, -21.5116) (64.0777, -21.518) (63.9866, -21.5246) (63.8955, -21.5315) (63.8046, -21.5388) (63.7138, -21.5464) (63.623, -21.5543) (63.5324, -21.5625) (63.4418, -21.571) (63.3514, -21.5799) (63.261, -21.5891) (63.1708, -21.5986) (63.0806, -21.6084) (62.9906, -21.6186) (62.9007, -21.6291) (62.8108, -21.64) (62.7211, -21.6512) (62.6315, -21.6627) (62.542, -21.6746) (62.4527, -21.6869) (62.3634, -21.6995) (62.2743, -21.7125) (62.1853, -21.7258) (62.0964, -21.7395) (62.0076, -21.7536) (61.919, -21.768) (61.8305, -21.7829) (61.7422, -21.7981) (61.654, -21.8137) (61.5731, -21.8284) (61.5099, -21.8401) (61.4644, -21.8487) (61.4364, -21.8541) (61.4261, -21.8561) knots -1 -1 -1 -1 -1 -1 -0.985714 -0.971429 -0.957143 -0.942857 -0.928571 -0.914286 -0.9 -0.885714 -0.871429 -0.857143 -0.842857 -0.828571 -0.814286 -0.8 -0.785714 -0.771429 -0.757143 -0.742857 -0.728571 -0.714286 -0.7 -0.685714 -0.671429 -0.657143 -0.642857 -0.628571 -0.614286 -0.6 -0.585714 -0.571429 -0.557143 -0.542857 -0.528571 -0.514286 -0.5 -0.485714 -0.471429 -0.457143 -0.442857 -0.428571 -0.414286 -0.405839 -0.405839 -0.405839 -0.405839 -0.405839 -0.405839
  arc A14 (61.4261, -21.8561) -> (60.836, -20.6774) centre (-2.0032, -52.8695) ccw
  spline S14 degree 5 poles (60.836, -20.6774) (60.8439, -20.6703) (60.8649, -20.6511) (60.8991, -20.6198) (60.9463, -20.5763) (61.0066, -20.5203) (61.0719, -20.4591) (61.137, -20.3975) (61.202, -20.3355) (61.2666, -20.2732) (61.3311, -20.2106) (61.3953, -20.1477) (61.4593, -20.0844) (61.5231, -20.0208) (61.5867, -19.9569) (61.6501, -19.8927) (61.7132, -19.8282) (61.7762, -19.7634) (61.8389, -19.6983) (61.9014, -19.6329) (61.9637, -19.5672) (62.0258, -19.5012) (62.0877, -19.435) (62.1494, -19.3684) (62.2109, -19.3016) (62.2722, -19.2345) (62.3333, -19.1671) (62.3942, -19.0995) (62.4549, -19.0316) (62.5154, -18.9634) (62.5757, -18.8949) (62.6359, -18.8262) (62.6958, -18.7573) (62.7555, -18.6881) (62.815, -18.6186) (62.8744, -18.5489) (62.9335, -18.4789) (62.9925, -18.4087) (63.0512, -18.3382) (63.1098, -18.2675) (63.1682, -18.1965) (63.2264, -18.1253) (63.2844, -18.0539) (63.3307, -17.9966) (63.3653, -17.9535) (63.3883, -17.9247) (63.3998, -17.9103) knots 0.405839 0.405839 0.405839 0.405839 0.405839 0.405839 0.414286 0.428571 0.442857 0.457143 0.471429 0.485714 0.5 0.514286 0.528571 0.542857 0.557143 0.571429 0.585714 0.6 0.614286 0.628571 0.642857 0.657143 0.671429 0.685714 0.7 0.714286 0.728571 0.742857 0.757143 0.771429 0.785714 0.8 0.814286 0.828571 0.842857 0.857143 0.871429 0.885714 0.9 0.914286 0.928571 0.942857 0.957143 0.971429 0.985714 1 1 1 1 1 1
  arc A15 (63.3998, -17.9103) -> (62.7659, -16.7493) centre (-2.0032, -52.8695) ccw
  spline S15 degree 5 poles (62.7659, -16.7493) (62.7476, -16.7512) (62.7109, -16.755) (62.6559, -16.7608) (62.5827, -16.7687) (62.4912, -16.7789) (62.3999, -16.7894) (62.3086, -16.8002) (62.2174, -16.8112) (62.1264, -16.8226) (62.0354, -16.8342) (61.9446, -16.8461) (61.8539, -16.8583) (61.7632, -16.8709) (61.6727, -16.8837) (61.5823, -16.8968) (61.492, -16.9102) (61.4018, -16.924) (61.3118, -16.938) (61.2218, -16.9523) (61.132, -16.967) (61.0423, -16.982) (60.9527, -16.9973) (60.8632, -17.0129) (60.7739, -17.0288) (60.6847, -17.0451) (60.5956, -17.0616) (60.5066, -17.0785) (60.4178, -17.0958) (60.3291, -17.1134) (60.2406, -17.1313) (60.1522, -17.1495) (60.0639, -17.1681) (59.9758, -17.1871) (59.8878, -17.2063) (59.8, -17.226) (59.7123, -17.246) (59.6248, -17.2664) (59.5374, -17.2871) (59.4502, -17.3082) (59.3631, -17.3297) (59.2763, -17.3516) (59.1966, -17.372) (59.1345, -17.3882) (59.0897, -17.4) (59.0622, -17.4074) (59.052, -17.4101) knots -1 -1 -1 -1 -1 -1 -0.985714 -0.971429 -0.957143 -0.942857 -0.928571 -0.914286 -0.9 -0.885714 -0.871429 -0.857143 -0.842857 -0.828571 -0.814286 -0.8 -0.785714 -0.771429 -0.757143 -0.742857 -0.728571 -0.714286 -0.7 -0.685714 -0.671429 -0.657143 -0.642857 -0.628571 -0.614286 -0.6 -0.585714 -0.571429 -0.557143 -0.542857 -0.528571 -0.514286 -0.5 -0.485714 -0.471429 -0.457143 -0.442857 -0.428571 -0.414286 -0.405839 -0.405839 -0.405839 -0.405839 -0.405839 -0.405839
  arc A16 (59.052, -17.4101) -> (58.3794, -16.2765) centre (-2.0032, -52.8695) ccw
  spline S16 degree 5 poles (58.3794, -16.2765) (58.3867, -16.2688) (58.4063, -16.2482) (58.4381, -16.2146) (58.4822, -16.1678) (58.5383, -16.1077) (58.5991, -16.0419) (58.6596, -15.9758) (58.72, -15.9094) (58.78, -15.8427) (58.8399, -15.7756) (58.8994, -15.7082) (58.9588, -15.6406) (59.0179, -15.5726) (59.0767, -15.5043) (59.1354, -15.4358) (59.1937, -15.3669) (59.2519, -15.2978) (59.3098, -15.2284) (59.3675, -15.1587) (59.425, -15.0887) (59.4822, -15.0185) (59.5393, -14.9479) (59.5961, -14.8772) (59.6526, -14.8061) (59.709, -14.7348) (59.7651, -14.6633) (59.821, -14.5914) (59.8767, -14.5194) (59.9322, -14.4471) (59.9875, -14.3745) (60.0425, -14.3017) (60.0974, -14.2286) (60.152, -14.1553) (60.2065, -14.0818) (60.2607, -14.008) (60.3147, -13.934) (60.3685, -13.8597) (60.4221, -13.7852) (60.4754, -13.7105) (60.5286, -13.6356) (60.5816, -13.5604) (60.6344, -13.485) (60.6764, -13.4246) (60.7079, -13.3791) (60.7288, -13.3487) (60.7392, -13.3335) knots 0.405839 0.405839 0.405839 0.405839 0.405839 0.405839 0.414286 0.428571 0.442857 0.457143 0.471429 0.485714 0.5 0.514286 0.528571 0.542857 0.557143 0.571429 0.585714 0.6 0.614286 0.628571 0.642857 0.657143 0.671429 0.685714 0.7 0.714286 0.728571 0.742857 0.757143 0.771429 0.785714 0.8 0.814286 0.828571 0.842857 0.857143 0.871429 0.885714 0.9 0.914286 0.928571 0.942857 0.957143 0.971429 0.985714 1 1 1 1 1 1
  arc A17 (60.7392, -13.3335) -> (60.0241, -12.2208) centre (-2.0032, -52.8695) ccw
  spline S17 degree 5 poles (60.0241, -12.2208) (60.0059, -12.224) (59.9696, -12.2304) (59.9152, -12.2401) (59.8427, -12.2532) (59.7522, -12.2699) (59.6618, -12.2869) (59.5716, -12.3041) (59.4815, -12.3216) (59.3914, -12.3394) (59.3016, -12.3575) (59.2118, -12.3759) (59.1222, -12.3946) (59.0327, -12.4135) (58.9433, -12.4328) (58.854, -12.4523) (58.7649, -12.4721) (58.676, -12.4923) (58.5871, -12.5127) (58.4984, -12.5334) (58.4099, -12.5545) (58.3215, -12.5758) (58.2332, -12.5974) (58.1451, -12.6194) (58.0571, -12.6417) (57.9693, -12.6642) (57.8816, -12.6871) (57.7941, -12.7103) (57.7067, -12.7339) (57.6195, -12.7577) (57.5325, -12.7819) (57.4456, -12.8064) (57.3589, -12.8313) (57.2723, -12.8564) (57.1859, -12.882) (57.0997, -12.9078) (57.0137, -12.934) (56.9278, -12.9606) (56.8422, -12.9875) (56.7567, -13.0148) (56.6714, -13.0424) (56.5863, -13.0704) (56.5083, -13.0965) (56.4475, -13.1171) (56.4037, -13.1321) (56.3768, -13.1414) (56.3668, -13.1448) knots -1 -1 -1 -1 -1 -1 -0.985714 -0.971429 -0.957143 -0.942857 -0.928571 -0.914286 -0.9 -0.885714 -0.871429 -0.857143 -0.842857 -0.828571 -0.814286 -0.8 -0.785714 -0.771429 -0.757143 -0.742857 -0.728571 -0.714286 -0.7 -0.685714 -0.671429 -0.657143 -0.642857 -0.628571 -0.614286 -0.6 -0.585714 -0.571429 -0.557143 -0.542857 -0.528571 -0.514286 -0.5 -0.485714 -0.471429 -0.457143 -0.442857 -0.428571 -0.414286 -0.405839 -0.405839 -0.405839 -0.405839 -0.405839 -0.405839
  arc A18 (56.3668, -13.1448) -> (55.615, -12.0621) centre (-2.0032, -52.8695) ccw
  spline S18 degree 5 poles (55.615, -12.0621) (55.6217, -12.0539) (55.6398, -12.032) (55.6692, -11.9961) (55.7098, -11.9463) (55.7614, -11.8824) (55.8174, -11.8124) (55.8731, -11.7422) (55.9285, -11.6716) (55.9837, -11.6008) (56.0386, -11.5296) (56.0932, -11.4582) (56.1476, -11.3864) (56.2017, -11.3144) (56.2555, -11.2421) (56.3091, -11.1696) (56.3624, -11.0967) (56.4155, -11.0236) (56.4683, -10.9502) (56.5209, -10.8766) (56.5732, -10.8027) (56.6253, -10.7286) (56.6772, -10.6542) (56.7288, -10.5795) (56.7801, -10.5046) (56.8313, -10.4295) (56.8821, -10.3541) (56.9328, -10.2785) (56.9832, -10.2026) (57.0334, -10.1265) (57.0833, -10.0502) (57.1331, -9.9736) (57.1826, -9.8969) (57.2318, -9.8198) (57.2809, -9.7426) (57.3297, -9.6651) (57.3783, -9.5875) (57.4266, -9.5096) (57.4748, -9.4315) (57.5227, -9.3531) (57.5704, -9.2746) (57.6179, -9.1958) (57.6651, -9.1169) (57.7027, -9.0535) (57.7309, -9.006) (57.7496, -8.9742) (57.7589, -8.9583) knots 0.405839 0.405839 0.405839 0.405839 0.405839 0.405839 0.414286 0.428571 0.442857 0.457143 0.471429 0.485714 0.5 0.514286 0.528571 0.542857 0.557143 0.571429 0.585714 0.6 0.614286 0.628571 0.642857 0.657143 0.671429 0.685714 0.7 0.714286 0.728571 0.742857 0.757143 0.771429 0.785714 0.8 0.814286 0.828571 0.842857 0.857143 0.871429 0.885714 0.9 0.914286 0.928571 0.942857 0.957143 0.971429 0.985714 1 1 1 1 1 1
  arc A19 (57.7589, -8.9583) -> (56.9662, -7.8993) centre (-2.0032, -52.8695) ccw
  spline S19 degree 5 poles (56.9662, -7.8993) (56.9483, -7.9038) (56.9126, -7.9128) (56.859, -7.9264) (56.7876, -7.9447) (56.6985, -7.9678) (56.6096, -7.9911) (56.5208, -8.0148) (56.4321, -8.0387) (56.3436, -8.0629) (56.2553, -8.0873) (56.167, -8.1121) (56.079, -8.1371) (55.991, -8.1624) (55.9033, -8.1879) (55.8157, -8.2138) (55.7282, -8.2399) (55.6409, -8.2664) (55.5537, -8.2931) (55.4667, -8.3201) (55.3799, -8.3474) (55.2932, -8.3749) (55.2067, -8.4028) (55.1204, -8.431) (55.0342, -8.4595) (54.9483, -8.4883) (54.8624, -8.5174) (54.7768, -8.5468) (54.6913, -8.5765) (54.606, -8.6065) (54.5209, -8.6368) (54.436, -8.6675) (54.3513, -8.6984) (54.2668, -8.7297) (54.1824, -8.7613) (54.0983, -8.7933) (54.0144, -8.8256) (53.9306, -8.8582) (53.8471, -8.8911) (53.7638, -8.9244) (53.6807, -8.9581) (53.5978, -8.9921) (53.5219, -9.0236) (53.4627, -9.0486) (53.42, -9.0667) (53.3938, -9.0778) (53.3841, -9.082) knots -1 -1 -1 -1 -1 -1 -0.985714 -0.971429 -0.957143 -0.942857 -0.928571 -0.914286 -0.9 -0.885714 -0.871429 -0.857143 -0.842857 -0.828571 -0.814286 -0.8 -0.785714 -0.771429 -0.757143 -0.742857 -0.728571 -0.714286 -0.7 -0.685714 -0.671429 -0.657143 -0.642857 -0.628571 -0.614286 -0.6 -0.585714 -0.571429 -0.557143 -0.542857 -0.528571 -0.514286 -0.5 -0.485714 -0.471429 -0.457143 -0.442857 -0.428571 -0.414286 -0.405839 -0.405839 -0.405839 -0.405839 -0.405839 -0.405839
  arc A20 (53.3841, -9.082) -> (52.557, -8.0556) centre (-2.0032, -52.8695) ccw
  spline S20 degree 5 poles (52.557, -8.0556) (52.5632, -8.047) (52.5796, -8.0238) (52.6064, -7.986) (52.6433, -7.9334) (52.6903, -7.8659) (52.7411, -7.7922) (52.7917, -7.7181) (52.8419, -7.6438) (52.8919, -7.5692) (52.9416, -7.4943) (52.9909, -7.4191) (53.04, -7.3437) (53.0889, -7.268) (53.1374, -7.1921) (53.1857, -7.1159) (53.2337, -7.0394) (53.2814, -6.9627) (53.3289, -6.8857) (53.3761, -6.8085) (53.423, -6.7311) (53.4696, -6.6534) (53.516, -6.5755) (53.5622, -6.4974) (53.6081, -6.419) (53.6537, -6.3404) (53.6991, -6.2616) (53.7442, -6.1826) (53.7891, -6.1033) (53.8337, -6.0238) (53.8781, -5.9441) (53.9222, -5.8642) (53.9661, -5.7841) (54.0098, -5.7037) (54.0532, -5.6232) (54.0963, -5.5425) (54.1393, -5.4615) (54.1819, -5.3804) (54.2244, -5.299) (54.2666, -5.2175) (54.3086, -5.1357) (54.3503, -5.0538) (54.3918, -4.9717) (54.4248, -4.9058) (54.4495, -4.8563) (54.4659, -4.8233) (54.4741, -4.8068) knots 0.405839 0.405839 0.405839 0.405839 0.405839 0.405839 0.414286 0.428571 0.442857 0.457143 0.471429 0.485714 0.5 0.514286 0.528571 0.542857 0.557143 0.571429 0.585714 0.6 0.614286 0.628571 0.642857 0.657143 0.671429 0.685714 0.7 0.714286 0.728571 0.742857 0.757143 0.771429 0.785714 0.8 0.814286 0.828571 0.842857 0.857143 0.871429 0.885714 0.9 0.914286 0.928571 0.942857 0.957143 0.971429 0.985714 1 1 1 1 1 1
  arc A21 (54.4741, -4.8068) -> (53.6078, -3.8071) centre (-2.0032, -52.8695) ccw
  spline S21 degree 5 poles (53.6078, -3.8071) (53.5903, -3.8128) (53.5553, -3.8244) (53.5028, -3.8417) (53.4329, -3.865) (53.3457, -3.8944) (53.2587, -3.9241) (53.1718, -3.954) (53.0851, -3.9842) (52.9985, -4.0146) (52.9121, -4.0453) (52.8259, -4.0763) (52.7398, -4.1075) (52.6539, -4.139) (52.5682, -4.1708) (52.4826, -4.2028) (52.3973, -4.2351) (52.3121, -4.2677) (52.227, -4.3006) (52.1422, -4.3337) (52.0575, -4.3671) (51.9731, -4.4008) (51.8888, -4.4348) (51.8047, -4.4691) (51.7207, -4.5036) (51.637, -4.5385) (51.5535, -4.5736) (51.4702, -4.6091) (51.3871, -4.6448) (51.3041, -4.6808) (51.2214, -4.7171) (51.1389, -4.7538) (51.0566, -4.7907) (50.9745, -4.8279) (50.8927, -4.8655) (50.811, -4.9033) (50.7296, -4.9415) (50.6484, -4.98) (50.5674, -5.0189) (50.4867, -5.058) (50.4062, -5.0975) (50.326, -5.1374) (50.2525, -5.1742) (50.1952, -5.2033) (50.1539, -5.2244) (50.1286, -5.2374) (50.1192, -5.2422) knots -1 -1 -1 -1 -1 -1 -0.985714 -0.971429 -0.957143 -0.942857 -0.928571 -0.914286 -0.9 -0.885714 -0.871429 -0.857143 -0.842857 -0.828571 -0.814286 -0.8 -0.785714 -0.771429 -0.757143 -0.742857 -0.728571 -0.714286 -0.7 -0.685714 -0.671429 -0.657143 -0.642857 -0.628571 -0.614286 -0.6 -0.585714 -0.571429 -0.557143 -0.542857 -0.528571 -0.514286 -0.5 -0.485714 -0.471429 -0.457143 -0.442857 -0.428571 -0.414286 -0.405839 -0.405839 -0.405839 -0.405839 -0.405839 -0.405839
  arc A22 (50.1192, -5.2422) -> (49.221, -4.2775) centre (-2.0032, -52.8695) ccw
  spline S22 degree 5 poles (49.221, -4.2775) (49.2265, -4.2685) (49.2413, -4.2442) (49.2653, -4.2045) (49.2984, -4.1495) (49.3404, -4.0788) (49.3859, -4.0016) (49.431, -3.9241) (49.4758, -3.8464) (49.5203, -3.7684) (49.5645, -3.6902) (49.6084, -3.6117) (49.652, -3.533) (49.6953, -3.454) (49.7383, -3.3748) (49.781, -3.2953) (49.8235, -3.2156) (49.8656, -3.1357) (49.9074, -3.0556) (49.949, -2.9752) (49.9903, -2.8946) (50.0313, -2.8138) (50.072, -2.7328) (50.1125, -2.6515) (50.1527, -2.5701) (50.1926, -2.4885) (50.2322, -2.4066) (50.2716, -2.3245) (50.3107, -2.2423) (50.3495, -2.1598) (50.3881, -2.0771) (50.4264, -1.9943) (50.4645, -1.9112) (50.5023, -1.828) (50.5398, -1.7446) (50.5771, -1.661) (50.6142, -1.5772) (50.651, -1.4932) (50.6875, -1.409) (50.7238, -1.3246) (50.7598, -1.2401) (50.7956, -1.1554) (50.8311, -1.0705) (50.8594, -1.0025) (50.8804, -0.9514) (50.8944, -0.9173) (50.9014, -0.9002) knots 0.405839 0.405839 0.405839 0.405839 0.405839 0.405839 0.414286 0.428571 0.442857 0.457143 0.471429 0.485714 0.5 0.514286 0.528571 0.542857 0.557143 0.571429 0.585714 0.6 0.614286 0.628571 0.642857 0.657143 0.671429 0.685714 0.7 0.714286 0.728571 0.742857 0.757143 0.771429 0.785714 0.8 0.814286 0.828571 0.842857 0.857143 0.871429 0.885714 0.9 0.914286 0.928571 0.942857 0.957143 0.971429 0.985714 1 1 1 1 1 1
  arc A23 (50.9014, -0.9002) -> (49.9661, 0.0351) centre (-2.0032, -52.8695) ccw
  spline S23 degree 5 poles (49.9661, 0.0351) (49.949, 0.0282) (49.9149, 0.0142) (49.8638, -0.0069) (49.7957, -0.0351) (49.7109, -0.0707) (49.6261, -0.1065) (49.5416, -0.1425) (49.4573, -0.1788) (49.3731, -0.2153) (49.2891, -0.2521) (49.2053, -0.2891) (49.1217, -0.3264) (49.0383, -0.364) (48.955, -0.4018) (48.872, -0.4398) (48.7891, -0.4782) (48.7065, -0.5167) (48.624, -0.5556) (48.5417, -0.5947) (48.4597, -0.6341) (48.3778, -0.6737) (48.2962, -0.7136) (48.2147, -0.7538) (48.1335, -0.7942) (48.0525, -0.835) (47.9717, -0.876) (47.8911, -0.9173) (47.8107, -0.9588) (47.7306, -1.0007) (47.6506, -1.0428) (47.571, -1.0852) (47.4915, -1.1279) (47.4123, -1.1709) (47.3333, -1.2142) (47.2546, -1.2578) (47.1761, -1.3017) (47.0978, -1.3459) (47.0199, -1.3904) (46.9421, -1.4353) (46.8647, -1.4804) (46.7875, -1.5259) (46.7168, -1.5679) (46.6617, -1.601) (46.6221, -1.625) (46.5978, -1.6397) (46.5887, -1.6452) knots -1 -1 -1 -1 -1 -1 -0.985714 -0.971429 -0.957143 -0.942857 -0.928571 -0.914286 -0.9 -0.885714 -0.871429 -0.857143 -0.842857 -0.828571 -0.814286 -0.8 -0.785714 -0.771429 -0.757143 -0.742857 -0.728571 -0.714286 -0.7 -0.685714 -0.671429 -0.657143 -0.642857 -0.628571 -0.614286 -0.6 -0.585714 -0.571429 -0.557143 -0.542857 -0.528571 -0.514286 -0.5 -0.485714 -0.471429 -0.457143 -0.442857 -0.428571 -0.414286 -0.405839 -0.405839 -0.405839 -0.405839 -0.405839 -0.405839
  arc A24 (46.5887, -1.6452) -> (45.624, -0.747) centre (-2.0032, -52.8695) ccw
  spline S24 degree 5 poles (45.624, -0.747) (45.6289, -0.7376) (45.6419, -0.7123) (45.663, -0.6711) (45.692, -0.6138) (45.7289, -0.5403) (45.7687, -0.4601) (45.8082, -0.3796) (45.8474, -0.2988) (45.8862, -0.2179) (45.9247, -0.1367) (45.9629, -0.0553) (46.0008, 0.0264) (46.0383, 0.1083) (46.0756, 0.1903) (46.1125, 0.2726) (46.1491, 0.3551) (46.1855, 0.4379) (46.2215, 0.5208) (46.2572, 0.6039) (46.2926, 0.6872) (46.3278, 0.7708) (46.3626, 0.8545) (46.3972, 0.9384) (46.4314, 1.0225) (46.4654, 1.1068) (46.4991, 1.1913) (46.5326, 1.2759) (46.5657, 1.3608) (46.5986, 1.4458) (46.6311, 1.531) (46.6635, 1.6164) (46.6955, 1.7019) (46.7273, 1.7877) (46.7588, 1.8735) (46.79, 1.9596) (46.821, 2.0458) (46.8517, 2.1322) (46.8821, 2.2188) (46.9123, 2.3055) (46.9422, 2.3924) (46.9718, 2.4794) (47.0012, 2.5666) (47.0245, 2.6365) (47.0419, 2.689) (47.0534, 2.724) (47.0592, 2.7416) knots 0.405839 0.405839 0.405839 0.405839 0.405839 0.405839 0.414286 0.428571 0.442857 0.457143 0.471429 0.485714 0.5 0.514286 0.528571 0.542857 0.557143 0.571429 0.585714 0.6 0.614286 0.628571 0.642857 0.657143 0.671429 0.685714 0.7 0.714286 0.728571 0.742857 0.757143 0.771429 0.785714 0.8 0.814286 0.828571 0.842857 0.857143 0.871429 0.885714 0.9 0.914286 0.928571 0.942857 0.957143 0.971429 0.985714 1 1 1 1 1 1
  arc A25 (47.0592, 2.7416) -> (46.0595, 3.6078) centre (-2.0032, -52.8695) ccw
  spline S25 degree 5 poles (46.0595, 3.6078) (46.043, 3.5996) (46.0099, 3.5832) (45.9605, 3.5586) (45.8946, 3.5255) (45.8125, 3.484) (45.7305, 3.4423) (45.6488, 3.4003) (45.5672, 3.3581) (45.4859, 3.3157) (45.4047, 3.273) (45.3238, 3.2301) (45.2431, 3.1869) (45.1625, 3.1435) (45.0822, 3.0999) (45.0021, 3.056) (44.9222, 3.0118) (44.8425, 2.9675) (44.763, 2.9228) (44.6837, 2.878) (44.6047, 2.8328) (44.5258, 2.7874) (44.4472, 2.7418) (44.3689, 2.6959) (44.2907, 2.6498) (44.2128, 2.6034) (44.1352, 2.5567) (44.0577, 2.5098) (43.9805, 2.4626) (43.9036, 2.4151) (43.8269, 2.3674) (43.7504, 2.3194) (43.6742, 2.2711) (43.5983, 2.2226) (43.5226, 2.1738) (43.4471, 2.1247) (43.372, 2.0753) (43.2971, 2.0256) (43.2225, 1.9757) (43.1481, 1.9254) (43.0741, 1.8749) (43.0003, 1.824) (42.9329, 1.7771) (42.8803, 1.7401) (42.8425, 1.7134) (42.8193, 1.6969) (42.8106, 1.6908) knots -1 -1 -1 -1 -1 -1 -0.985714 -0.971429 -0.957143 -0.942857 -0.928571 -0.914286 -0.9 -0.885714 -0.871429 -0.857143 -0.842857 -0.828571 -0.814286 -0.8 -0.785714 -0.771429 -0.757143 -0.742857 -0.728571 -0.714286 -0.7 -0.685714 -0.671429 -0.657143 -0.642857 -0.628571 -0.614286 -0.6 -0.585714 -0.571429 -0.557143 -0.542857 -0.528571 -0.514286 -0.5 -0.485714 -0.471429 -0.457143 -0.442857 -0.428571 -0.414286 -0.405839 -0.405839 -0.405839 -0.405839 -0.405839 -0.405839
  arc A26 (42.8106, 1.6908) -> (41.7843, 2.5179) centre (-2.0032, -52.8695) ccw
  spline S26 degree 5 poles (41.7843, 2.5179) (41.7885, 2.5276) (41.7996, 2.5537) (41.8177, 2.5964) (41.8426, 2.6556) (41.8742, 2.7315) (41.9082, 2.8144) (41.9418, 2.8975) (41.9751, 2.9808) (42.0081, 3.0644) (42.0407, 3.1481) (42.073, 3.232) (42.1049, 3.3162) (42.1365, 3.4005) (42.1678, 3.485) (42.1988, 3.5698) (42.2295, 3.6547) (42.2598, 3.7398) (42.2898, 3.8251) (42.3195, 3.9105) (42.3489, 3.9962) (42.378, 4.082) (42.4068, 4.168) (42.4353, 4.2541) (42.4634, 4.3405) (42.4913, 4.427) (42.5189, 4.5136) (42.5462, 4.6005) (42.5732, 4.6875) (42.5999, 4.7746) (42.6263, 4.8619) (42.6525, 4.9494) (42.6783, 5.037) (42.7039, 5.1248) (42.7292, 5.2127) (42.7542, 5.3008) (42.7789, 5.389) (42.8034, 5.4774) (42.8276, 5.5659) (42.8515, 5.6545) (42.8751, 5.7433) (42.8985, 5.8323) (42.9216, 5.9213) (42.9399, 5.9927) (42.9534, 6.0463) (42.9624, 6.0821) (42.9669, 6.0999) knots 0.405839 0.405839 0.405839 0.405839 0.405839 0.405839 0.414286 0.428571 0.442857 0.457143 0.471429 0.485714 0.5 0.514286 0.528571 0.542857 0.557143 0.571429 0.585714 0.6 0.614286 0.628571 0.642857 0.657143 0.671429 0.685714 0.7 0.714286 0.728571 0.742857 0.757143 0.771429 0.785714 0.8 0.814286 0.828571 0.842857 0.857143 0.871429 0.885714 0.9 0.914286 0.928571 0.942857 0.957143 0.971429 0.985714 1 1 1 1 1 1
  arc A27 (42.9669, 6.0999) -> (41.908, 6.8927) centre (-2.0032, -52.8695) ccw
  spline S27 degree 5 poles (41.908, 6.8927) (41.8921, 6.8833) (41.8603, 6.8646) (41.8127, 6.8365) (41.7494, 6.7988) (41.6704, 6.7516) (41.5917, 6.7041) (41.5131, 6.6564) (41.4348, 6.6085) (41.3567, 6.5604) (41.2788, 6.512) (41.2011, 6.4634) (41.1237, 6.4146) (41.0464, 6.3656) (40.9694, 6.3163) (40.8926, 6.2668) (40.8161, 6.2171) (40.7397, 6.1671) (40.6636, 6.1169) (40.5878, 6.0665) (40.5122, 6.0159) (40.4368, 5.965) (40.3616, 5.9139) (40.2867, 5.8625) (40.2121, 5.8109) (40.1377, 5.7591) (40.0635, 5.707) (39.9896, 5.6546) (39.916, 5.6021) (39.8426, 5.5492) (39.7695, 5.4962) (39.6967, 5.4428) (39.6241, 5.3892) (39.5518, 5.3354) (39.4798, 5.2813) (39.4081, 5.2269) (39.3367, 5.1723) (39.2655, 5.1174) (39.1946, 5.0623) (39.1241, 5.0069) (39.0538, 4.9512) (38.9839, 4.8952) (38.9199, 4.8435) (38.8701, 4.8029) (38.8343, 4.7736) (38.8123, 4.7555) (38.8042, 4.7487) knots -1 -1 -1 -1 -1 -1 -0.985714 -0.971429 -0.957143 -0.942857 -0.928571 -0.914286 -0.9 -0.885714 -0.871429 -0.857143 -0.842857 -0.828571 -0.814286 -0.8 -0.785714 -0.771429 -0.757143 -0.742857 -0.728571 -0.714286 -0.7 -0.685714 -0.671429 -0.657143 -0.642857 -0.628571 -0.614286 -0.6 -0.585714 -0.571429 -0.557143 -0.542857 -0.528571 -0.514286 -0.5 -0.485714 -0.471429 -0.457143 -0.442857 -0.428571 -0.414286 -0.405839 -0.405839 -0.405839 -0.405839 -0.405839 -0.405839
  arc A28 (38.8042, 4.7487) -> (37.7214, 5.5005) centre (-2.0032, -52.8695) ccw